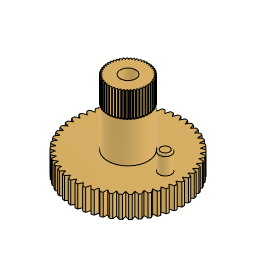
MG996R_Gear_4 v5 (Autodesk Fusion 360 design; units mm, degrees)
Autodesk Fusion 360 part; units mm, degrees
sketch "Sketch1" plane through (0, 0, 0) normal (0, 0, 1) x (1, 0, 0)
  circle A0 centre (0, 0) radius 8.9
  circle A1 centre (0, 0) radius 3.25
  dimension "d1" = 17.8
  dimension "d2" = 6.5
  constraint coincident A0.centre A1.centre
  measures "d1" diameter of A0
  measures "d2" diameter of A1
extrude "Extrude1" add sketch "Sketch1" along normal blind 3.5
sketch "Sketch2" plane through (0, 0, 0) normal (0, 0, -1) x (1, 0, 0)
  circle A0 centre (0, 0) radius 3.25
  circle A1 centre (0, 0) radius 8.9
  circle A2 centre (0, 0) radius 6
  circle A3 centre (0, 0) radius 5
  dimension "d5" = 12
  dimension "d6" = 10
  constraint coincident A0.centre A1.centre
  measures "d5" diameter of A2
  measures "d6" diameter of A3
extrude "Extrude2" add sketch "Sketch2" along normal blind 1 contours A2
extrude "Extrude3" add sketch "Sketch1" along normal blind 14 contours A1
sketch "Sketch4" plane through (0, 0, 14) normal (0, 0, 1) x (-1, 0, 0)
  circle A0 centre (0, 0) radius 3.25
  circle A1 centre (0, 0) radius 1.25
  dimension "d11" = 2.5
  constraint concentric A0 A1
  measures "d11" diameter of A1
extrude "Extrude4" cut sketch "Sketch4" against normal blind 37 contours A1
extrude "Extrude5" cut 1 faces at (3.7314, 0.2484, 0) along direction (0, 0, 1) blind 1.5
sketch "Sketch5" plane through (0, 0, 14) normal (0, 0, 1) x (-1, 0, 0)
  circle A0 centre (0, 0) radius 1.25
  circle A1 centre (0, 0) radius 3.25
  circle A2 centre (0, 0) radius 3.25
  line L0 (0.15, -3.2465) -> (0, -2.9867)
  line L1 (0, -2.9867) -> (-0.15, -3.2465)
  dimension "d16" = 0.3
  dimension "d17" = 0.3
  constraint concentric A0 A2
  constraint coincident A2 L0.start
  constraint coincident A2 L1.end
  constraint equal L0 L1
  constraint equal A1 A2
  constraint vertical A0.centre L0.end
  measures "d16" distance of L0.start L0.end
  measures "d17" distance of L0.start L1.end
extrude "Extrude6" cut sketch "Sketch5" against normal blind 4 contours A1 A2 L0 L1 picked at (0, -3.162)
pattern_circular "C-Pattern1" count 50 over 360 about axis through (0, 0, 14) along (0, 0, -1) of "Extrude6"
sketch "Sketch6" plane through (0, 0, 3.5) normal (0, 0, 1) x (-1, 0, 0)
  circle A0 centre (0, 0) radius 3.25
  circle A1 centre (0, 0) radius 8.9
  circle A2 centre (0, 0) radius 8.9
  line L0 (0.35, -8.8931) -> (0, -8.2869)
  line L1 (0, -8.2869) -> (-0.35, -8.8931)
  dimension "d22" = 0.7
  dimension "d23" = 0.7
  dimension "d24" = 0.7
  constraint coincident A0.centre A1.centre
  constraint coincident A2 L0.start
  constraint coincident A2 L1.end
  constraint equal A1 A2
  constraint vertical A0.centre L0.end
  measures "d22" distance of L0.start L0.end
  measures "d23" distance of L0.end L1.end
  measures "d24" horizontal distance of L0.start L1.end
extrude "Extrude7" cut sketch "Sketch6" against normal blind 6.5 contours A1 A2 L0 L1 picked at (0, -8.6951)
pattern_circular "C-Pattern2" count 50 over 360 about axis through (0, 0, 14) along (0, 0, -1) of "Extrude7"
sketch "Sketch7" plane through (0, 0, 3.5) normal (0, 0, 1) x (-1, 0, 0)
  line L0 (1.0386, -8.2216) -> (1.4618, -8.7791)
  arc A0 (1.4618, -8.7791) -> (1.8726, -8.7008) centre (0, 0) ccw
  line L1 (1.8726, -8.7008) -> (2.0609, -8.0265)
  line L2 (2.0609, -8.0265) -> (2.5506, -8.5267)
  arc A1 (2.5506, -8.5267) -> (2.9484, -8.3975) centre (0, 0) ccw
  line L3 (2.9484, -8.3975) -> (3.0506, -7.705)
  line L4 (3.0506, -7.705) -> (3.5992, -8.1398)
  arc A2 (3.5992, -8.1398) -> (3.9776, -7.9617) centre (0, 0) ccw
  line L5 (3.9776, -7.9617) -> (3.9922, -7.2619)
  line L6 (3.9922, -7.2619) -> (4.591, -7.6245)
  arc A3 (4.591, -7.6245) -> (4.9441, -7.4004) centre (0, 0) ccw
  line L7 (4.9441, -7.4004) -> (4.8709, -6.7042)
  line L8 (4.8709, -6.7042) -> (5.5104, -6.989)
  arc A4 (5.5104, -6.989) -> (5.8326, -6.7224) centre (0, 0) ccw
  line L9 (5.8326, -6.7224) -> (5.6728, -6.0409)
  line L10 (5.6728, -6.0409) -> (6.3429, -6.2432)
  arc A5 (6.3429, -6.2432) -> (6.6292, -5.9384) centre (0, 0) ccw
  line L11 (6.6292, -5.9384) -> (6.3852, -5.2823)
  line L12 (6.3852, -5.2823) -> (7.0754, -5.399)
  arc A6 (7.0754, -5.399) -> (7.3212, -5.0607) centre (0, 0) ccw
  line L13 (7.3212, -5.0607) -> (6.9969, -4.4403)
  line L14 (6.9969, -4.4403) -> (7.6962, -4.4697)
  arc A7 (7.6962, -4.4697) -> (7.8977, -4.1032) centre (0, 0) ccw
  line L15 (7.8977, -4.1032) -> (7.4982, -3.5284)
  line L16 (7.4982, -3.5284) -> (8.1958, -3.4698)
  arc A8 (8.1958, -3.4698) -> (8.3497, -3.081) centre (0, 0) ccw
  line L17 (8.3497, -3.081) -> (7.8813, -2.5608)
  line L18 (7.8813, -2.5608) -> (8.566, -2.4153)
  arc A9 (8.566, -2.4153) -> (8.67, -2.0102) centre (0, 0) ccw
  line L19 (8.67, -2.0102) -> (8.1401, -1.5528)
  line L20 (8.1401, -1.5528) -> (8.8012, -1.3226)
  arc A10 (8.8012, -1.3226) -> (8.8536, -0.9077) centre (0, 0) ccw
  line L21 (8.8536, -0.9077) -> (8.2705, -0.5203)
  line L22 (8.2705, -0.5203) -> (8.8975, -0.2091)
  arc A11 (8.8975, -0.2091) -> (8.8975, 0.2091) centre (0, 0) ccw
  line L23 (8.8975, 0.2091) -> (8.2705, 0.5203)
  line L24 (8.2705, 0.5203) -> (8.8536, 0.9077)
  arc A12 (8.8536, 0.9077) -> (8.8012, 1.3226) centre (0, 0) ccw
  line L25 (8.8012, 1.3226) -> (8.1401, 1.5528)
  line L26 (8.1401, 1.5528) -> (8.67, 2.0102)
  arc A13 (8.67, 2.0102) -> (8.566, 2.4153) centre (0, 0) ccw
  line L27 (8.566, 2.4153) -> (7.8813, 2.5608)
  line L28 (7.8813, 2.5608) -> (8.3497, 3.081)
  arc A14 (8.3497, 3.081) -> (8.1958, 3.4698) centre (0, 0) ccw
  line L29 (8.1958, 3.4698) -> (7.4982, 3.5284)
  line L30 (7.4982, 3.5284) -> (7.8977, 4.1032)
  arc A15 (7.8977, 4.1032) -> (7.6962, 4.4697) centre (0, 0) ccw
  line L31 (7.6962, 4.4697) -> (6.9969, 4.4403)
  line L32 (6.9969, 4.4403) -> (7.3212, 5.0607)
  arc A16 (7.3212, 5.0607) -> (7.0754, 5.399) centre (0, 0) ccw
  line L33 (7.0754, 5.399) -> (6.3852, 5.2823)
  line L34 (6.3852, 5.2823) -> (6.6292, 5.9384)
  arc A17 (6.6292, 5.9384) -> (6.3429, 6.2432) centre (0, 0) ccw
  line L35 (6.3429, 6.2432) -> (5.6728, 6.0409)
  line L36 (5.6728, 6.0409) -> (5.8326, 6.7224)
  arc A18 (5.8326, 6.7224) -> (5.5104, 6.989) centre (0, 0) ccw
  line L37 (5.5104, 6.989) -> (4.8709, 6.7042)
  line L38 (4.8709, 6.7042) -> (4.9441, 7.4004)
  arc A19 (4.9441, 7.4004) -> (4.591, 7.6245) centre (0, 0) ccw
  line L39 (4.591, 7.6245) -> (3.9922, 7.2619)
  line L40 (3.9922, 7.2619) -> (3.9776, 7.9617)
  arc A20 (3.9776, 7.9617) -> (3.5992, 8.1398) centre (0, 0) ccw
  line L41 (3.5992, 8.1398) -> (3.0506, 7.705)
  line L42 (3.0506, 7.705) -> (2.9484, 8.3975)
  arc A21 (2.9484, 8.3975) -> (2.5506, 8.5267) centre (0, 0) ccw
  line L43 (2.5506, 8.5267) -> (2.0609, 8.0265)
  line L44 (2.0609, 8.0265) -> (1.8726, 8.7008)
  arc A22 (1.8726, 8.7008) -> (1.4618, 8.7791) centre (0, 0) ccw
  line L45 (1.4618, 8.7791) -> (1.0386, 8.2216)
  line L46 (1.0386, 8.2216) -> (0.7674, 8.8669)
  arc A23 (0.7674, 8.8669) -> (0.35, 8.8931) centre (0, 0) ccw
  line L47 (0.35, 8.8931) -> (0, 8.2869)
  line L48 (0, 8.2869) -> (-0.35, 8.8931)
  arc A24 (-0.35, 8.8931) -> (-0.7674, 8.8669) centre (0, 0) ccw
  line L49 (-0.7674, 8.8669) -> (-1.0386, 8.2216)
  line L50 (-1.0386, 8.2216) -> (-1.4618, 8.7791)
  arc A25 (-1.4618, 8.7791) -> (-1.8726, 8.7008) centre (0, 0) ccw
  line L51 (-1.8726, 8.7008) -> (-2.0609, 8.0265)
  line L52 (-2.0609, 8.0265) -> (-2.5506, 8.5267)
  arc A26 (-2.5506, 8.5267) -> (-2.9484, 8.3975) centre (0, 0) ccw
  line L53 (-2.9484, 8.3975) -> (-3.0506, 7.705)
  line L54 (-3.0506, 7.705) -> (-3.5992, 8.1398)
  arc A27 (-3.5992, 8.1398) -> (-3.9776, 7.9617) centre (0, 0) ccw
  line L55 (-3.9776, 7.9617) -> (-3.9922, 7.2619)
  line L56 (-3.9922, 7.2619) -> (-4.591, 7.6245)
  arc A28 (-4.591, 7.6245) -> (-4.9441, 7.4004) centre (0, 0) ccw
  line L57 (-4.9441, 7.4004) -> (-4.8709, 6.7042)
  line L58 (-4.8709, 6.7042) -> (-5.5104, 6.989)
  arc A29 (-5.5104, 6.989) -> (-5.8326, 6.7224) centre (0, 0) ccw
  line L59 (-5.8326, 6.7224) -> (-5.6728, 6.0409)
  line L60 (-5.6728, 6.0409) -> (-6.3429, 6.2432)
  arc A30 (-6.3429, 6.2432) -> (-6.6292, 5.9384) centre (0, 0) ccw
  line L61 (-6.6292, 5.9384) -> (-6.3852, 5.2823)
  line L62 (-6.3852, 5.2823) -> (-7.0754, 5.399)
  arc A31 (-7.0754, 5.399) -> (-7.3212, 5.0607) centre (0, 0) ccw
  line L63 (-7.3212, 5.0607) -> (-6.9969, 4.4403)
  line L64 (-6.9969, 4.4403) -> (-7.6962, 4.4697)
  arc A32 (-7.6962, 4.4697) -> (-7.8977, 4.1032) centre (0, 0) ccw
  line L65 (-7.8977, 4.1032) -> (-7.4982, 3.5284)
  line L66 (-7.4982, 3.5284) -> (-8.1958, 3.4698)
  arc A33 (-8.1958, 3.4698) -> (-8.3497, 3.081) centre (0, 0) ccw
  line L67 (-8.3497, 3.081) -> (-7.8813, 2.5608)
  line L68 (-7.8813, 2.5608) -> (-8.566, 2.4153)
  arc A34 (-8.566, 2.4153) -> (-8.67, 2.0102) centre (0, 0) ccw
  line L69 (-8.67, 2.0102) -> (-8.1401, 1.5528)
  line L70 (-8.1401, 1.5528) -> (-8.8012, 1.3226)
  arc A35 (-8.8012, 1.3226) -> (-8.8536, 0.9077) centre (0, 0) ccw
  line L71 (-8.8536, 0.9077) -> (-8.2705, 0.5203)
  line L72 (-8.2705, 0.5203) -> (-8.8975, 0.2091)
  arc A36 (-8.8975, 0.2091) -> (-8.8975, -0.2091) centre (0, 0) ccw
  line L73 (-8.8975, -0.2091) -> (-8.2705, -0.5203)
  line L74 (-8.2705, -0.5203) -> (-8.8536, -0.9077)
  arc A37 (-8.8536, -0.9077) -> (-8.8012, -1.3226) centre (0, 0) ccw
  line L75 (-8.8012, -1.3226) -> (-8.1401, -1.5528)
  line L76 (-8.1401, -1.5528) -> (-8.67, -2.0102)
  arc A38 (-8.67, -2.0102) -> (-8.566, -2.4153) centre (0, 0) ccw
  line L77 (-8.566, -2.4153) -> (-7.8813, -2.5608)
  line L78 (-7.8813, -2.5608) -> (-8.3497, -3.081)
  arc A39 (-8.3497, -3.081) -> (-8.1958, -3.4698) centre (0, 0) ccw
  line L79 (-8.1958, -3.4698) -> (-7.4982, -3.5284)
  line L80 (-7.4982, -3.5284) -> (-7.8977, -4.1032)
  arc A40 (-7.8977, -4.1032) -> (-7.6962, -4.4697) centre (0, 0) ccw
  line L81 (-7.6962, -4.4697) -> (-6.9969, -4.4403)
  line L82 (-6.9969, -4.4403) -> (-7.3212, -5.0607)
  arc A41 (-7.3212, -5.0607) -> (-7.0754, -5.399) centre (0, 0) ccw
  line L83 (-7.0754, -5.399) -> (-6.3852, -5.2823)
  line L84 (-6.3852, -5.2823) -> (-6.6292, -5.9384)
  arc A42 (-6.6292, -5.9384) -> (-6.3429, -6.2432) centre (0, 0) ccw
  line L85 (-6.3429, -6.2432) -> (-5.6728, -6.0409)
  line L86 (-5.6728, -6.0409) -> (-5.8326, -6.7224)
  arc A43 (-5.8326, -6.7224) -> (-5.5104, -6.989) centre (0, 0) ccw
  line L87 (-5.5104, -6.989) -> (-4.8709, -6.7042)
  line L88 (-4.8709, -6.7042) -> (-4.9441, -7.4004)
  arc A44 (-4.9441, -7.4004) -> (-4.591, -7.6245) centre (0, 0) ccw
  line L89 (-4.591, -7.6245) -> (-3.9922, -7.2619)
  line L90 (-3.9922, -7.2619) -> (-3.9776, -7.9617)
  arc A45 (-3.9776, -7.9617) -> (-3.5992, -8.1398) centre (0, 0) ccw
  line L91 (-3.5992, -8.1398) -> (-3.0506, -7.705)
  line L92 (-3.0506, -7.705) -> (-2.9484, -8.3975)
  arc A46 (-2.9484, -8.3975) -> (-2.5506, -8.5267) centre (0, 0) ccw
  line L93 (-2.5506, -8.5267) -> (-2.0609, -8.0265)
  line L94 (-2.0609, -8.0265) -> (-1.8726, -8.7008)
  arc A47 (-1.8726, -8.7008) -> (-1.4618, -8.7791) centre (0, 0) ccw
  line L95 (-1.4618, -8.7791) -> (-1.0386, -8.2216)
  line L96 (-1.0386, -8.2216) -> (-0.7674, -8.8669)
  arc A48 (-0.7674, -8.8669) -> (-0.35, -8.8931) centre (0, 0) ccw
  line L97 (-0.35, -8.8931) -> (0, -8.2869)
  line L98 (0, -8.2869) -> (0.35, -8.8931)
  arc A49 (0.35, -8.8931) -> (0.7674, -8.8669) centre (0, 0) ccw
  line L99 (0.7674, -8.8669) -> (1.0386, -8.2216)
  circle A50 centre (0, 0) radius 3.25
  circle A51 centre (-6, 0) radius 1
  dimension "d29" = 2
  dimension "d30" = 6
  measures "d29" diameter of A51
  measures "d30" distance of A0.centre A51.centre
extrude "Extrude8" add sketch "Sketch7" along normal blind 3 contours A51
fillet "Fillet1" radius 0.3 1 edges at (6.9323, 0.3616, 6.5)
sketch "Sketch8" plane through (0, 0, 1.5) normal (0, 0, -1) x (1, 0, 0)
  circle A0 centre (0, 0) radius 1.25
  circle A1 centre (0, 0) radius 5
  line L0 (-1.5, -1) -> (1.5, -1)
  arc A2 (1.5, -1) -> (1.5, 1) centre (1.5, 0) ccw
  line L1 (1.5, 1) -> (-1.5, 1)
  arc A3 (-1.5, 1) -> (-1.5, -1) centre (-1.5, 0) ccw
  line L2 (-1.5, 0) -> (1.5, 0) construction
  dimension "d35" = 2
  dimension "d36" = 3
  constraint tangent L0 A2
  constraint tangent A2 L1
  constraint parallel L0 L1
  constraint tangent L1 A3
  constraint tangent L0 A3
  constraint horizontal L2
  constraint coincident A0.centre A1.centre
  constraint midpoint L2 A0.centre
  measures "d35" distance of L0 L1
  measures "d36" distance of A3.centre A2.centre
extrude "Extrude9" cut sketch "Sketch8" against normal blind 4 contours A0 L0 A2 L1 | A0 L0 L1 A3
